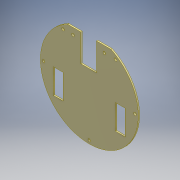
# Autodesk Inventor part: Tapa
Saved by Autodesk Inventor 2016 (Build 200138000, 138)
## iProperties
Created: 2019-03-15
Part Number: Tapa
Material: Nilón 6/6
Document SubType Name: Modeling
Designer: FIMCP
Mass: 34.2037 g
Surface Area: 318.751 cm^2
Volume: 30.2688 cm^3
Density: 1.13 g/cm^3
Appearance: Nilón 6
Author: FIMCP
Autodesk Inventor part; units mm, degrees
ref_plane "YZ Plane" through (0, 0, 0) normal (1, 0, 0) x (0, 1, 0)
ref_plane "XZ Plane" through (0, 0, 0) normal (0, 1, 0) x (-1, 0, 0)
ref_plane "XY Plane" through (0, 0, 0) normal (0, 0, 1) x (1, 0, 0)
sketch "Boceto1" plane through (0, 0, 0) normal (0, 1, 0) x (-1, 0, 0)
  arc A0 (-18, 72.808) -> (20, 72.2842) centre (0, 0) ccw
  line L0 (-18, 72.808) -> (-18, 72.2842)
  line L1 (-11, 25) -> (13, 25)
  line L2 (55, 0) -> (40, 0)
  line L3 (40, 0) -> (40, -38)
  line L4 (40, -38) -> (55, -38)
  line L5 (55, -38) -> (55, 0)
  line L6 (-40, 0) -> (-55, 0)
  line L7 (-55, 0) -> (-55, -38)
  line L8 (-55, -38) -> (-40, -38)
  line L9 (-40, -38) -> (-40, 0)
  line L10 (20, 72.2842) -> (13, 72.2842)
  line L11 (13, 72.2842) -> (13, 25)
  line L12 (-18, 72.808) -> (-11, 72.808)
  line L13 (-11, 72.808) -> (-11, 25)
  line L14 (-18, 72.2842) -> (-18, 72.808)
  dimension "d0" = 150
  dimension "d1" = 18
  dimension "d2" = 25
  dimension "d3" = 15
  dimension "d4" = 38
  dimension "d5" = 15
  dimension "d6" = 38
  dimension "d7" = 40
  dimension "d8" = 40
  constraints: 30 end point, 5 parallel, 4 horizontal, 4 perpendicular, 2 point on circle, 1 centre point, 1 coincident, 1 point on line
  measures "d0" diameter of A0
  measures "d1" distance from line of L0 point (0, 0)
  measures "d2" distance from line of L1 point (0, 0)
  measures "d3" distance of L4.end L4.start
  measures "d4" distance of L4.start L2.end
  measures "d5" distance of L9.start L8.start
  measures "d6" distance of L8.start L6.end
  measures "d7" distance from line of L9 point (0, 0)
  measures "d8" distance from line of L3 point (0, 0)
extrude "Extrusión1" add sketch "Boceto1" along normal blind 2
sketch "Boceto2" plane through (0, 0, 0) normal (0, 1, 0) x (-1, 0, 0)
  line L0 (-74.7999, 67.2842) -> (80.1068, 67.2842)
  line L1 (80.1068, 67.2842) -> (80.1068, 81.1614)
  line L2 (80.1068, 81.1614) -> (-74.7999, 81.1614)
  line L3 (-74.7999, 81.1614) -> (-74.7999, 67.2842)
  line L4 (20, 72.2842) -> (13, 72.2842) projected
  point P0 (0, 0)
  dimension "d13" = 5
  constraints: 8 end point, 2 parallel, 1 horizontal, 1 perpendicular
  measures "d13" distance between parallel lines of L4 L0
extrude "Extrusión2" cut sketch "Boceto2" along normal blind 2
sketch "Boceto3" plane through (0, 0, 0) normal (0, 1, 0) x (-1, 0, 0)
  circle A0 centre (-70, 0) radius 2
  circle A1 centre (0, -70) radius 2
  circle A2 centre (70, 0) radius 2
  point P0 (0, 0)
  dimension "d14" = 4
  dimension "d15" = 4
  dimension "d16" = 4
  dimension "d17" = 70
  dimension "d18" = 70
  dimension "d19" = 70
  constraints: 3 centre point
  measures "d14" diameter of A0
  measures "d15" diameter of A1
  measures "d16" diameter of A2
  measures "d17" distance of A0.centre point (0, 0)
  measures "d18" distance of A2.centre point (0, 0)
  measures "d19" distance of A1.centre point (0, 0)
extrude "Extrusión3" cut sketch "Boceto3" along normal mid plane 6
sketch "Boceto6" plane through (0, 0, 0) normal (0, 1, 0) x (-1, 0, 0)
  line L0 (-27, 57.2842) -> (-36.2309, 57.2842)
  arc A0 (-43.4373, 54.8927) -> (-36.2309, 57.2842) centre (-40.2309, 57.2842) ccw
  arc A1 (-27, 57.2842) -> (-23, 53.2842) centre (-23, 57.2842) ccw
  circle A2 centre (-23, 57.2842) radius 2
  arc A3 (25, 53.2842) -> (29, 57.2842) centre (25, 57.2842) ccw
  circle A4 centre (25, 57.2842) radius 2
  arc A5 (36.2309, 57.2842) -> (43.4373, 54.8927) centre (40.2309, 57.2842) ccw
  circle A6 centre (40.2309, 57.2842) radius 2
  circle A7 centre (-40.2309, 57.2842) radius 2
  point P0 (0, 0)
  dimension "d22" = 4
  dimension "d23" = 4
  dimension "d24" = 4
  dimension "d25" = 4
  constraints: 8 centre point, 8 point on circle, 4 coincident, 2 end point
  measures "d22" diameter of A2
  measures "d23" diameter of A4
  measures "d24" diameter of A6
  measures "d25" diameter of A7
extrude "Extrusión4" cut sketch "Boceto6" along normal mid plane 6
